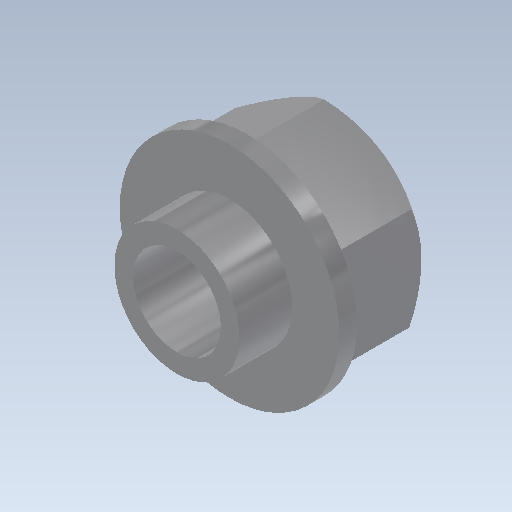
# Autodesk Inventor part: Eccentric Spacer
Saved by Autodesk Inventor 2020.3 (Build 243373000, 373)
## iProperties
Created: 2016-04-09
Part Number: Eccentric Spacer
Material: Generic
Document SubType Name: Modeling
Designer: Ben
Density: 1 g/cm^3
Appearance: Default
Author: Ben
Autodesk Inventor part; units mm, degrees
ref_plane "YZ Plane" through (0, 0, 0) normal (1, 0, 0) x (0, 1, 0)
ref_plane "XZ Plane" through (0, 0, 0) normal (0, 1, 0) x (-1, 0, 0)
ref_plane "XY Plane" through (0, 0, 0) normal (0, 0, 1) x (1, 0, 0)
sketch "Sketch1" plane through (0, 0, 0) normal (0, 0, 1) x (1, 0, 0)
  line L0 (5, -2.8868) -> (0, -5.7735)
  line L1 (0, -5.7735) -> (-5, -2.8868)
  line L2 (-5, -2.8868) -> (-5, 2.8868)
  line L3 (-5, 2.8868) -> (0, 5.7735)
  line L4 (0, 5.7735) -> (5, 2.8868)
  line L5 (5, 2.8868) -> (5, -2.8868)
  point P0 (0, 0)
  point P1 (0, 0)
  dimension "d0" = 10
  constraints: 12 end point, 1 coincident, 13 other
  measures "d0" distance between parallel lines of L5 L2
extrude "Extrusion1" add sketch "Sketch1" along normal blind 5
sketch "Sketch2" plane through (0, 0, 5) normal (0, 0, 1) x (1, 0, 0)
  circle A0 centre (0, 0) radius 6.25
  dimension "d3" = 12.5
  constraints: 1 centre point, 1 coincident
  measures "d3" diameter of A0
extrude "Extrusion2" add sketch "Sketch2" along normal blind 1
sketch "Sketch3" plane through (0, 0, 6) normal (0, 0, 1) x (1, 0, 0)
  circle A0 centre (0, 0) radius 6.25 projected
  circle A1 centre (0, 0) radius 3.56
  dimension "d6" = 7.12
  constraints: 1 centre point, 1 coincident
  measures "d6" diameter of A1
extrude "Extrusion3" add sketch "Sketch3" along normal blind 3 contours A1
sketch "Sketch4" plane through (0, 0, 9) normal (0, 0, 1) x (1, 0, 0)
  circle A0 centre (0, 0) radius 3.56 projected
  circle A1 centre (0, 0) radius 2.5
  dimension "d9" = 5
  constraints: 1 centre point, 1 coincident
  measures "d9" diameter of A1
extrude "Extrusion4" cut sketch "Sketch4" against normal up to next contours A1
sketch "Sketch5" plane through (0, 0, 0) normal (1, 0, 0) x (0, 1, 0)
  arc A0 (0.1187, -1.552) -> (0.1187, 15.367) centre (0.1187, 6.9075) ccw
  arc A1 (0.1187, -2.8398) -> (0.1187, 16.6548) centre (0.1187, 6.9075) ccw
  line L0 (0.1187, -2.8398) -> (0.1187, 16.6548)
  point P0 (0, 0)
  constraints: 4 point on circle, 2 centre point, 2 end point, 2 point on line, 1 coincident, 1 vertical
revolve "Revolution1" cut sketch "Sketch5" angle 360 about axis through (0, 0.1187, -2.8398) along (0, 0, 1) contours A0 L0 A1
body "Solid1"
